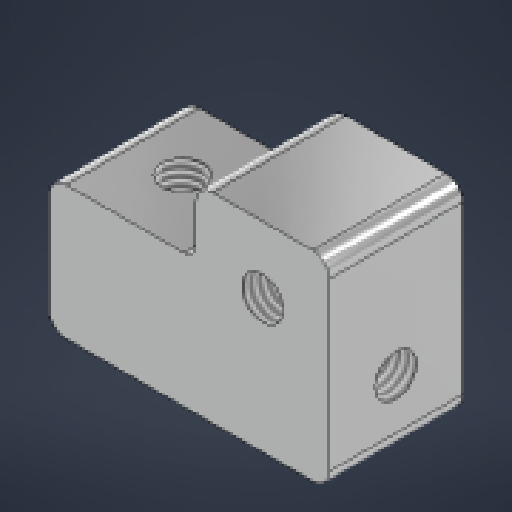
# Autodesk Inventor part: PLATE,NUT-BLOCK,L-SHAPE
Saved by Autodesk Inventor 2026 (Build 300175000, 175)
## iProperties
Created: 2026-02-08
Part Number: PLATE,NUT-BLOCK,L-SHAPE
Material: Aluminum 6061
Document SubType Name: Sheet Metal
Designer: Owen L
Mass: 12.4617 g
Surface Area: 23.0814 cm^2
Volume: 4.61546 cm^3
Density: 2.7 g/cm^3
Sheet Metal Rule: Default
Appearance: Aluminum - Flat
Author: Owen L
Autodesk Inventor part; units mm, degrees
ref_plane "YZ Plane" through (0, 0, 0) normal (1, 0, 0) x (0, 1, 0)
ref_plane "XZ Plane" through (0, 0, 0) normal (0, 1, 0) x (-1, 0, 0)
ref_plane "XY Plane" through (0, 0, 0) normal (0, 0, 1) x (1, 0, 0)
sketch "Sketch1" plane through (0, 0, 0) normal (0, 0, 1) x (1, 0, 0)
  line L0 (6.35, -9.525) -> (-6.35, -9.525)
  line L1 (-6.35, 3.175) -> (-6.35, 9.525)
  line L2 (-6.35, 9.525) -> (6.35, 9.525)
  line L3 (6.35, 9.525) -> (6.35, -9.525)
  line L4 (6.35, -9.525) -> (-6.35, 9.525) construction
  line L5 (-6.35, -9.525) -> (6.35, 9.525) construction
  line L6 (-6.35, -9.525) -> (-20.32, -9.525)
  line L7 (-20.32, -9.525) -> (-20.32, 3.175)
  line L8 (-20.32, 3.175) -> (-6.35, 3.175)
  line L9 (-6.35, 3.175) -> (-6.35, -9.525) construction
  point P0 (0, 0)
  dimension "d0" = 12.7
  dimension "d1" = 19.05
  dimension "d3" = 12.7
  dimension "d4" = 13.97
  measures "d0" distance of L1.end L2.end
  measures "d1" distance of L0.end L1.end
  measures "d3" distance of L6.end L7.end
  measures "d4" distance of L1.start L7.end
extrude "Plate1" add sketch "Sketch1" along normal blind 12.7
sketch "Sketch2" plane through (0, 0, 12.7) normal (0, 0, 1) x (1, 0, 0)
  line L0 (-6.35, 9.525) -> (6.35, 9.525) projected
  point P0 (0, 0)
  point P1 (0, 3.175)
  dimension "d5" = 6.35
  constraints: 1 vertical alignment
  measures "d5" distance from line of L0 point (0, 3.175)
hole "Hole1" at (0, 3.175, 12.7) direction (0, 0, -1) diameter 3.9624 depth 13.6144 tip angle 118 thread size "10-32 UNF" class "2B" standard "ANSI Unified Screw Threads"
sketch "Sketch3" plane through (-20.32, -9.525, 0) normal (0, -1, 0) x (1, 0, 0)
  line L0 (0, 0) -> (0, 12.7) projected
  line L1 (0, 0) -> (26.67, 0) projected
  point P0 (20.32, 0)
  point P1 (6.35, 6.35)
  dimension "d13" = 6.35
  dimension "d14" = 6.35
  measures "d13" distance from line of L0 point (6.35, 6.35)
  measures "d14" distance from line of L1 point (6.35, 6.35)
hole "Hole2" at (-13.97, -9.525, 6.35) direction (0, 1, 0) diameter 3.9624 depth 23.1394 tip angle 118 thread size "10-32 UNF" class "2B" standard "ANSI Unified Screw Threads"
sketch "Sketch4" plane through (6.35, -9.525, 0) normal (1, 0, 0) x (0, 0, -1)
  line L0 (0, 0) -> (-12.7, 0) projected
  line L1 (-12.7, 19.05) -> (-12.7, 0) projected
  point P0 (0, 9.525)
  point P1 (-6.35, 6.35)
  dimension "d22" = 6.35
  dimension "d23" = 6.35
  measures "d22" distance from line of L0 point (-6.35, 6.35)
  measures "d23" distance from line of L1 point (-6.35, 6.35)
hole "Hole3" at (6.35, -3.175, 6.35) direction (-1, 0, 0) diameter 3.9624 depth 12.7 tip angle 118 thread size "10-32 UNF" class "2B" standard "ANSI Unified Screw Threads"
fillet "Corner Round1" radius 1.5875 5 edges at (6.35, 9.525, 6.35) (-6.35, 9.525, 6.35) (-20.32, 3.175, 6.35) (-20.32, -9.525, 6.35) (6.35, -9.525, 6.35)
fillet "Corner Round1" radius 1.143 1 edges at (-6.35, 3.175, 6.35)
equation "\"d14\" = d13"
equation "\"d29\" = Thickness"
equation "\"d2\" = Thickness"
equation "\"BendRadius\" = Thickness"
equation "\"BendReliefWidth\" = Thickness"
equation "\"BendReliefDepth\" = 0.5 * Thickness"
equation "\"CornerReliefSize\" = 4 * Thickness"
equation "\"MinimumRemnant\" = 2 * Thickness"
equation "\"TransitionRadius\" = BendRadius"
equation "\"JacobiRadiusSize\" = BendRadius"
equation "\"GapSize\" = Thickness"
equation "\"Thickness\" = 12.7"
body "Solid1"
